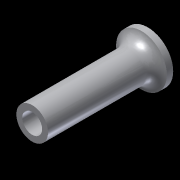
# Autodesk Inventor part: Pneumatic Standoff Curved
Saved by Autodesk Inventor 2014 SP1 (Build 180222100, 222)
## iProperties
Created: 2014-01-12
Part Number: Pneumatic Standoff Curved
Material: Aluminum 6061
Document SubType Name: Modeling
Designer: Rauhul Varma
Mass: 2.83431 g
Surface Area: 13.85 cm^2
Volume: 1.04587 cm^3
Density: 2.71 g/cm^3
Appearance: Aluminum - Flat
Author: Rauhul Varma
Autodesk Inventor part; units mm, degrees
ref_plane "YZ Plane" through (0, 0, 0) normal (1, 0, 0) x (0, 1, 0)
ref_plane "XZ Plane" through (0, 0, 0) normal (0, 1, 0) x (-1, 0, 0)
ref_plane "XY Plane" through (0, 0, 0) normal (0, 0, 1) x (1, 0, 0)
sketch "Sketch1" plane through (0, 0, 0) normal (0, 0, 1) x (1, 0, 0)
  circle A0 centre (0, 0) radius 6.35
  dimension "d0" = 12.7
  constraints: 1 centre point, 1 coincident
  measures "d0" diameter of A0
extrude "Extrusion1" add sketch "Sketch1" along normal blind 1.5875
sketch "Sketch2" plane through (0, 0, 1.5875) normal (0, 0, 1) x (1, 0, 0)
  circle A0 centre (0, 0) radius 6.35 projected
  circle A1 centre (0, 0) radius 3.9688
  dimension "d3" = 7.9375
  constraints: 1 centre point, 1 coincident
  measures "d3" diameter of A1
extrude "Extrusion2" add sketch "Sketch2" along normal blind 27.3495 contours A1
fillet "Fillet1" radius 3.175 1 edges at (-3.9688, 0, 1.5875)
sketch "Sketch3" plane through (0, 0, 28.937) normal (0, 0, 1) x (1, 0, 0)
  circle A0 centre (0, 0) radius 3.9687 projected
  constraints: 1 coincident
hole "Hole1" at (0, 0, 28.937) direction (0, 0, -1) diameter 4.9784 end through all clearance for "Flat Head Machine Screw (82)" size "#10" standard "Ansi Unified Screw Threads"
body "Solid1"
